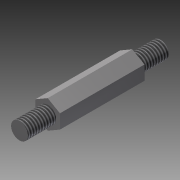
# Autodesk Inventor part: Heatbed_Standoff
Saved by Autodesk Inventor 2014 (Build 180170000, 170)
## iProperties
Created: 2013-12-17
Part Number: Heatbed_Standoff
Material: Stainless Steel
Document SubType Name: Modeling
Designer: Bram
Density: 8.08 g/cm^3
Appearance: Semi-Polished
Author: Bram
Autodesk Inventor part; units mm, degrees
ref_plane "YZ Plane" through (0, 0, 0) normal (1, 0, 0) x (0, 1, 0)
ref_plane "XZ Plane" through (0, 0, 0) normal (0, 1, 0) x (-1, 0, 0)
ref_plane "XY Plane" through (0, 0, 0) normal (0, 0, 1) x (1, 0, 0)
sketch "Sketch1" plane through (0, 0, 0) normal (0, 1, 0) x (-1, 0, 0)
  circle A0 centre (0, 0) radius 1.5
  dimension "d0" = 3
  constraints: 1 centre point, 1 coincident
  measures "d0" diameter of A0
extrude "Extrusion1" add sketch "Sketch1" along normal blind 5
sketch "Sketch2" plane through (0, 5, 0) normal (0, 1, 0) x (1, 0, 0)
  circle A0 centre (0, 0) radius 1.5 projected
  circle A1 centre (0, 0) radius 2.5
  line L0 (0, 2.5) -> (2.1651, 1.25)
  line L1 (2.1651, 1.25) -> (2.1651, -1.25)
  line L2 (2.1651, -1.25) -> (0, -2.5)
  line L3 (0, -2.5) -> (-2.1651, -1.25)
  line L4 (-2.1651, -1.25) -> (-2.1651, 1.25)
  line L5 (-2.1651, 1.25) -> (0, 2.5)
  dimension "d5" = 5
  constraints: 12 end point, 2 coincident, 1 vertical alignment, 15 other
extrude "Extrusion2" add sketch "Sketch2" along normal blind 15 contours A0 | L1 L2 L3 L4 L5 L0
sketch "Sketch3" plane through (0, 20, 0) normal (0, 1, 0) x (1, 0, 0)
  circle A0 centre (0, 0) radius 1.5
  dimension "d8" = 3
  constraints: 1 centre point, 1 coincident
  measures "d8" diameter of A0
extrude "Extrusion3" add sketch "Sketch3" along normal blind 5
thread "Thread1" size "M3x0.5" class "6g" standard "ANSI Metric M Profile" full length
thread "Thread2" size "M3x0.5" class "6g" standard "ANSI Metric M Profile" full length
body "Solid1"
